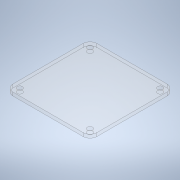
# Autodesk Inventor part: oled_cover
Saved by Autodesk Inventor 2020.2 (Build 242310000, 310)
## iProperties
Created: 2020-04-12
Part Number: oled_cover
Material: PMMA Plastic
Document SubType Name: Modeling
Designer: agmlego
Mass: 2.75358 g
Surface Area: 32.0391 cm^2
Volume: 2.31783 cm^3
Density: 1.188 g/cm^3
Appearance: Polycarbonate - Clear
Author: agmlego
Autodesk Inventor part; units mm, degrees
ref_plane "YZ Plane" through (0, 0, 0) normal (1, 0, 0) x (0, 1, 0)
ref_plane "XZ Plane" through (0, 0, 0) normal (0, 1, 0) x (-1, 0, 0)
ref_plane "XY Plane" through (0, 0, 0) normal (0, 0, 1) x (1, 0, 0)
sketch "Sketch1" plane through (0, 0, 0) normal (0, 1, 0) x (-1, 0, 0)
  line L0 (3.175, 0) -> (35.3816, 0)
  line L1 (38.5566, -3.175) -> (38.5566, -35.3816)
  line L2 (35.3816, -38.5566) -> (3.175, -38.5566)
  line L3 (0, -35.3816) -> (0, -3.175)
  arc A0 (38.5566, -3.175) -> (35.3816, 0) centre (35.3816, -3.175) ccw
  arc A1 (3.175, 0) -> (0, -3.175) centre (3.175, -3.175) ccw
  arc A2 (0, -35.3816) -> (3.175, -38.5566) centre (3.175, -35.3816) ccw
  arc A3 (35.3816, -38.5566) -> (38.5566, -35.3816) centre (35.3816, -35.3816) ccw
  line L4 (35.3816, -3.175) -> (3.175, -35.3816) construction
  point P0 (0, 0)
  dimension "d0" = 3.175
  dimension "d5" = 45.547
  constraints: 10 end point, 8 point on circle, 8 tangent, 4 centre point, 3 equal radius, 2 coincident, 2 parallel, 2 perpendicular, 2 point on line, 1 horizontal
  measures "d0" radius of A0
  measures "d5" distance of L4.start L4.end
extrude "Extrusion1" add sketch "Sketch1" along normal blind 1.5875
sketch "Sketch2" plane through (0, 1.5875, 0) normal (0, 1, 0) x (1, 0, 0)
  arc A0 (-38.5566, 3.175) -> (-35.3816, 0) centre (-35.3816, 3.175) ccw construction
  arc A1 (-35.3816, 38.5566) -> (-38.5566, 35.3816) centre (-35.3816, 35.3816) ccw construction
  arc A2 (0, 35.3816) -> (-3.175, 38.5566) centre (-3.175, 35.3816) ccw construction
  arc A3 (-3.175, 0) -> (0, 3.175) centre (-3.175, 3.175) ccw construction
  point P0 (0, 0)
  constraints: 4 coincident
hole "Hole1" at (-35.3816, 1.5875, -3.175) at (-35.3816, 1.5875, -35.3816) at (-3.175, 1.5875, -35.3816) at (-3.175, 1.5875, -3.175) direction (0, -1, 0) diameter 2.3876 end through all clearance for "Socket Head Cap Screw" size "M2" standard "Ansi Metric M Profile"
body "Solid1"
